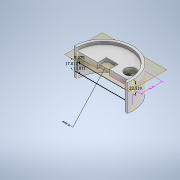
# Autodesk Inventor part: airframe
Saved by Autodesk Inventor 2022 (Build 260153000, 153)
## iProperties
Created: 2021-07-29
Part Number: airframe
Material: Generic
Document SubType Name: Modeling
Designer: WASHINGTON
Density: 1 g/cm^3
Appearance: Default
Author: WASHINGTON
Autodesk Inventor part; units mm, degrees
ref_plane "YZ Plane" through (0, 0, 0) normal (1, 0, 0) x (0, 1, 0)
ref_plane "XZ Plane" through (0, 0, 0) normal (0, 1, 0) x (-1, 0, 0)
ref_plane "XY Plane" through (0, 0, 0) normal (0, 0, 1) x (1, 0, 0)
sketch "Sketch1" plane through (0, 0, 0) normal (0, 1, 0) x (-1, 0, 0)
  arc A0 (-48.5586, 8.5622) -> (49.3077, 0) centre (0, 0) ccw construction
  line L0 (-25, -42.5) -> (25, -42.5) construction
  line L1 (25, -42.5) -> (25, 42.5) construction
  line L2 (25, 42.5) -> (-25, 42.5) construction
  line L3 (-25, -42.5) -> (25, 42.5) construction
  line L4 (25, -42.5) -> (-25, 42.5) construction
  arc A1 (-48.5586, 8.5622) -> (49.3077, 0) centre (0, 0) ccw
  arc A2 (-53.4827, 9.4304) -> (54.3077, 0) centre (0, 0) ccw
  line L5 (-48.5586, 8.5622) -> (-53.4827, 9.4304)
  line L6 (54.3077, 0) -> (49.3077, 0)
  dimension "d0" = 85
  dimension "d1" = 50
  dimension "d2" = 5
  dimension "d4" = 54.3077
  dimension "d5" = 59.535
  dimension "d6" = 170
  dimension "d7" = 42.5
  dimension "d8" = 0
  constraints: 14 end point, 6 point on circle, 3 centre point, 2 coincident, 2 horizontal, 2 midpoint, 1 concentric, 1 parallel, 1 perpendicular
  measures "d0" distance of L0.end L1.end
  measures "d1" distance of L0.start L0.end
  measures "d2" radial gap between concentric circles of A0 A2
  measures "d4" radius of A2
  measures "d5" angle of L6 L4
  measures "d6" angle of L6 L5
  measures "d7" distance between parallel lines of L6 L0
  measures "d8" distance from line of point (0, 0) L5
extrude "Extrusion1" add sketch "Sketch1" along normal blind 25 and the other way blind 25
sketch "Sketch2" plane through (0, 0, 0) normal (1, 0, 0) x (0, 1, 0)
  point P0 (0, 0)
sketch "Sketch3" plane through (0, 0, 0) normal (0, 0, 1) x (1, 0, 0)
  line L0 (11.5, -6) -> (-11.5, -6)
  line L1 (-11.5, -6) -> (-11.5, 6)
  line L2 (-11.5, 6) -> (11.5, 6)
  line L3 (11.5, 6) -> (11.5, -6)
  line L4 (11.5, -6) -> (-11.5, 6) construction
  line L5 (-11.5, -6) -> (11.5, 6) construction
  line L6 (15.5, 10) -> (-15.5, 10)
  line L7 (-15.5, 10) -> (-15.5, -10)
  line L8 (-15.5, -10) -> (15.5, -10)
  line L9 (15.5, -10) -> (15.5, 10)
  point P0 (0, 0)
  dimension "d11" = 23
  dimension "d12" = 12
  dimension "d13" = 4
  constraints: 20 end point, 4 parallel, 2 midpoint, 2 perpendicular, 1 horizontal, 3 other
  measures "d11" distance of L1.end L2.end
  measures "d12" distance of L0.start L2.end
  measures "d13" distance between parallel lines of L2 L6
extrude "Extrusion2" add sketch "Sketch3" against normal up to next
sketch "Sketch4" plane through (0, 0, 0) normal (0, 0, 1) x (1, 0, 0)
  line L0 (15.5, 10) -> (-15.5, 10) projected
  line L1 (-15.5, -10) -> (15.5, -10)
  line L2 (15.5, -10) -> (15.5, 10)
  line L3 (15.5, 10) -> (-15.5, 10)
  line L4 (-15.5, 10) -> (-15.5, -10)
  line L5 (-15.5, -10) -> (15.5, 10) construction
  line L6 (15.5, -10) -> (-15.5, 10) construction
  point P0 (0, 0)
  point P1 (-15.5, 10)
  constraints: 12 end point, 2 midpoint, 2 parallel, 1 horizontal, 1 perpendicular
extrude "Extrusion3" cut sketch "Sketch4" against normal blind 25
sketch "Sketch5" plane through (0, 0, 0) normal (0, 1, 0) x (-1, 0, 0)
  point P0 (0, 0)
sketch "Sketch6" plane through (0, 0, 0) normal (0, 0, 1) x (1, 0, 0)
  line L0 (-49.3077, -25) -> (-49.3077, 25) projected
  line L1 (-49.3077, 7.7599) -> (-49.3077, -14.5309)
  line L2 (53.4827, -25) -> (53.4827, 25) projected
  line L3 (53.4827, -14.5309) -> (-53.8854, -14.5309)
  line L4 (-49.3077, 2.4805) -> (53.4827, 2.4805)
  line L5 (53.4827, 2.4805) -> (53.4827, -14.5309)
  line L6 (-49.3077, -14.5309) -> (-49.3077, 2.4805)
  line L7 (48.7697, -14.5309) -> (48.5586, 2.4805)
  line L8 (48.5586, -25) -> (48.5586, 25) projected
  point P0 (0, 0)
  dimension "d24" = 17.0114
  dimension "d25" = 22.5195
  dimension "d26" = 5.2794
  dimension "d27" = 17.0114
  constraints: 12 end point, 6 point on line, 1 horizontal, 1 parallel
  measures "d24" distance between parallel lines of L4 L3
  measures "d25" distance from line of L2.end L4
  measures "d26" distance from line of L1.start L4
  measures "d27" distance from line of L1.end L4
chamfer "Chamfer1" distance 1 angle 45 1 edges at (0, -6, -25)
sketch "Sketch7" plane through (0, 0, 0) normal (0, 0, 1) x (1, 0, 0)
  line L0 (-15.5, 10) -> (48.5586, 10)
  line L1 (48.5586, 10) -> (48.5586, 20)
  line L2 (48.5586, -25) -> (48.5586, 25) projected
  line L3 (48.5586, 20) -> (-49.3077, 20)
  line L4 (-49.3077, 20) -> (-49.3077, 10)
  line L5 (-49.3077, -25) -> (-49.3077, 25) projected
  line L6 (-15.5, 10) -> (-49.3077, 10)
  point P0 (0, 0)
  dimension "d33" = 10
  constraints: 10 end point, 3 point on line, 2 horizontal, 1 perpendicular
  measures "d33" distance between parallel lines of L0 L3
extrude "Extrusion4" add sketch "Sketch7" against normal up to next
sketch "Sketch8" plane through (15.5, -10, -25) normal (1, 0, 0) x (0, 0, -1)
  line L0 (0, 20) -> (0, 0) projected
  line L1 (21.8081, 20) -> (21.8081, 0) projected
  line L2 (0, 11) -> (21.8081, 11)
  line L3 (21.8081, 11) -> (21.8081, 7)
  line L4 (21.8081, 7) -> (0, 7)
  line L5 (0, 7) -> (0, 11)
  point P0 (-25, 10)
  point P1 (0, 16)
  point P2 (0, 3)
  point P3 (0, 7)
  point P4 (21.8081, 11)
  dimension "d36" = 4
  dimension "d39" = 4
  constraints: 8 end point, 2 parallel, 2 point on line, 1 horizontal, 1 perpendicular
  measures "d36" distance of L4.end L2.start
  measures "d39" distance of point (0, 3) L4.end
extrude "Extrusion5" cut sketch "Sketch8" against normal up to surface (4 mm away)
sketch "Sketch9" plane through (-49.3077, 10, 0) normal (0, -1, 0) x (1, 0, 0)
  circle A0 centre (83.1273, -16.0011) radius 10
  point P0 (49.3077, 0)
  dimension "d42" = 20
  dimension "d43" = 37.4138
  constraints: 1 centre point
  measures "d42" diameter of A0
  measures "d43" distance of A0.centre point (49.308, 0)
extrude "Extrusion6" cut sketch "Sketch9" against normal up to next
sketch "Sketch10" plane through (0, 0, 0) normal (0, 1, 0) x (-1, 0, 0)
  point P0 (0, 0)
ref_plane "Work Plane1" through (-49.3077, 15, 0) normal (0, 1, 0) x (1, 0, 0)
sketch "Sketch11" plane through (-49.3077, 15, 0) normal (0, 1, 0) x (1, 0, 0)
  line L0 (60.1077, 0) -> (60.1077, 16)
  line L1 (60.1077, 16) -> (38.5077, 16)
  line L2 (38.5077, 16) -> (38.5077, 0)
  line L3 (38.5077, -16) -> (60.1077, 16) construction
  line L4 (60.1077, -16) -> (38.5077, 16) construction
  line L5 (97.8663, 0) -> (0, 0) projected
  line L6 (38.5077, 0) -> (60.1077, 0)
  point P0 (49.3077, 0)
  dimension "d47" = 32
  dimension "d48" = 21.6
  dimension "d49" = 124.019
  dimension "d50" = 55.981
  dimension "d51" = 16
  constraints: 12 end point, 2 midpoint, 2 parallel, 2 point on line, 1 vertical
  measures "d47" distance of L4.start L0.end
  measures "d48" distance of L0.end L1.end
  measures "d49" angle of L5 L4
  measures "d50" angle of L3 L5
  measures "d51" distance from line of L3.start L5
extrude "Extrusion7" cut sketch "Sketch11" along normal up to next
sketch "Sketch12" plane through (-49.3077, 15, 0) normal (0, 1, 0) x (1, 0, 0)
  line L0 (60.1077, 0) -> (38.5077, 0) projected
  line L1 (38.5077, 0) -> (38.5077, 16) projected
  line L2 (60.1077, 0) -> (38.5077, 0)
  line L3 (38.5077, 0) -> (38.5077, 4)
  line L4 (38.5077, 4) -> (60.1077, 4)
  line L5 (60.1077, 4) -> (60.1077, 0)
  point P0 (49.3077, 0)
  dimension "d54" = 4
  constraints: 8 end point, 2 parallel, 1 horizontal, 1 perpendicular, 1 point on line
  measures "d54" distance between parallel lines of L0 L4
extrude "Extrusion8" cut sketch "Sketch12" against normal up to next
sketch "Sketch13" plane through (-49.3077, 15, 0) normal (0, 1, 0) x (1, 0, 0)
  line L0 (38.5077, 4) -> (60.1077, 4) projected
  line L1 (60.1077, 16) -> (38.5077, 16) projected
  line L2 (60.1077, 4) -> (38.5077, 4)
  line L3 (38.5077, 4) -> (38.5077, 16)
  line L4 (38.5077, 16) -> (60.1077, 16)
  line L5 (60.1077, 16) -> (60.1077, 4)
  circle A0 centre (40.8077, 14) radius 1.25
  line L6 (49.3077, 16) -> (49.3077, 4) construction
  circle A1 centre (57.8077, 14) radius 1.25
  point P0 (49.3077, 0)
  dimension "d57" = 2.5
  dimension "d58" = 2.3
  dimension "d59" = 2
  constraints: 10 end point, 2 centre point, 2 midpoint, 2 parallel, 1 horizontal, 1 perpendicular, 1 symmetric about line, 1 other
  measures "d57" diameter of A0
  measures "d58" distance from line of L3 A0.centre
  measures "d59" distance from line of L1 A0.centre
extrude "Extrusion9" add sketch "Sketch13" along normal blind 5 contours A0 | A1
body "Solid1"
